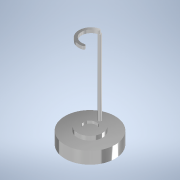
# Autodesk Inventor part: Robot-Axis5-Adapter
Saved by Autodesk Inventor 2021 (Build 250183000, 183)
## iProperties
Created: 2001-08-22
Part Number: Robot-Axis5-Adapter
Document SubType Name: ﾓﾃﾞﾘﾝｸﾞ
Designer: Administrator
Density: 1 g/cm^3
Material: Generic
Appearance: Black Chrome
Control State: 0
Master: False
Checked Out: False
Shininess: 21.0
Length Units: 11269
Angle Units: 11279
Time Units: 11290
Mass Units: 11283
Length Display Precision: 3
Angle Display Precision: 2
Density: 0.0
Volumn: 0.0
Area: 0.0
PropertySet Name: Model Information
Author: Administrator
Autodesk Inventor part; units mm, degrees
ref_plane "YZ Plane" through (0, 0, 0) normal (1, 0, 0) x (0, 1, 0)
ref_plane "XZ Plane" through (0, 0, 0) normal (0, 1, 0) x (-1, 0, 0)
ref_plane "XY Plane" through (0, 0, 0) normal (0, 0, 1) x (1, 0, 0)
sketch "ｽｹｯﾁ1" plane through (0, 0, 0) normal (0, 0, 1) x (1, 0, 0)
  circle A0 centre (0, 0) radius 40
  dimension "d0" = 80
  constraints: 1 centre point
  measures "d0" diameter of A0
extrude "Extrusion1" add sketch "ｽｹｯﾁ1" along normal blind 19.3
sketch "ｽｹｯﾁ2" plane through (0, 0, 19.3) normal (0, 0, 1) x (1, 0, 0)
  circle A0 centre (0, 0) radius 40 projected
  circle A1 centre (0, 0) radius 20
  dimension "d3" = 40
  constraints: 1 centre point, 1 coincident
  measures "d3" diameter of A1
extrude "Extrusion2" add sketch "ｽｹｯﾁ2" along normal blind 6.5 contours A1
sketch "ｽｹｯﾁ3" plane through (0, 0, 25.8) normal (0, 0, 1) x (1, 0, 0)
  circle A0 centre (0, 0) radius 20 projected
  circle A1 centre (0, 0) radius 10
  line L0 (0, 0) -> (0, 15.75)
  circle A2 centre (0, 15.75) radius 2.5
  dimension "d6" = 20
  dimension "d9" = 15.75
  dimension "d10" = 5
  constraints: 2 centre point, 2 coincident, 2 end point, 1 vertical
  measures "d6" diameter of A1
  measures "d9" distance of L0.start L0.end
  measures "d10" diameter of A2
extrude "Extrusion3" cut sketch "ｽｹｯﾁ3" against normal blind 4 contours A1 | A2
sketch "Sketch4" plane through (0, 0, 25.8) normal (0, 0, 1) x (1, 0, 0)
  circle A0 centre (0, 15.75) radius 2.5 projected
  circle A1 centre (0, 15.75) radius 2.5
  point P0 (0, 0)
  constraints: 1 centre point, 1 coincident
extrude "Extrusion4" add sketch "Sketch4" along normal blind 120
sketch "Sketch5" plane through (0, 15.75, 145.8) normal (0, 0, 1) x (1, 0, 0)
  arc A0 (-1.5175, -0.2348) -> (7.9156, -33.8904) centre (3.1807, -17.0678) ccw construction
  arc A1 (-2.1073, 1.8781) -> (8.51, -36.0021) centre (3.1807, -17.0678) ccw
  arc A2 (-0.9278, -2.3478) -> (7.3213, -31.7788) centre (3.1807, -17.0678) ccw
  arc A3 (-0.9278, -2.3478) -> (-2.1073, 1.8781) centre (-1.5175, -0.2348) ccw
  arc A4 (8.51, -36.0021) -> (7.3213, -31.7788) centre (7.9156, -33.8904) ccw
  point P0 (0, -15.75)
  constraints: 10 point on circle, 5 centre point, 4 tangent
extrude "Extrusion5" add sketch "Sketch5" along normal blind 5
body "Solid1"
